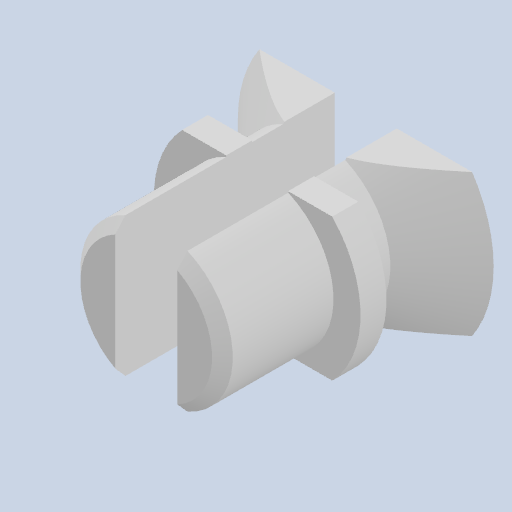
# Autodesk Inventor part: middle_gear_vtulka
Saved by Autodesk Inventor 2022 (Build 260153000, 153)
## iProperties
Created: 2024-12-03
Part Number: middle_gear_vtulka
Material: Типовые
Document SubType Name: Modeling
Designer: Andrey
Density: 1 g/cm^3
Appearance: По умолчанию
Author: Andrey
Autodesk Inventor part; units mm, degrees
ref_plane "YZ Plane" through (0, 0, 0) normal (1, 0, 0) x (0, 1, 0)
ref_plane "XZ Plane" through (0, 0, 0) normal (0, 1, 0) x (-1, 0, 0)
ref_plane "XY Plane" through (0, 0, 0) normal (0, 0, 1) x (1, 0, 0)
sketch "Эскиз1" plane through (0, 0, 0) normal (0, 1, 0) x (-1, 0, 0)
  line L0 (-19.5644, -4.2) -> (17.0679, -4.2) projected
  line L1 (-19.5644, -1.2) -> (17.0679, -1.2) projected
  line L2 (-4.6407, 3.8947) -> (-2.8372, 3.8947) projected
  line L3 (2.3395, 3.8947) -> (4.1648, 3.8947) projected
  line L4 (-7.157, -1) -> (5.9403, -1) projected
  line L5 (8.7851, 3.8947) -> (-8.7851, 3.8947)
  line L6 (4, 0) -> (-4, 0) projected
  line L7 (2.95, 0) -> (-2.95, 0)
  line L8 (2.95, -4.2) -> (2.95, 3.8947)
  line L9 (-2.95, -4.2) -> (-2.95, 3.8947)
  line L10 (2.95, -1.2) -> (4, -1.2)
  line L11 (4, 0) -> (4, -1.2)
  line L12 (-4, 0) -> (-4, -1.2)
  line L13 (-2.95, 3.8947) -> (-2.55, 4.2947)
  line L14 (-2.95, 3.8947) -> (-2.3843, 3.8947) construction
  line L15 (0, 4.2947) -> (-2.55, 4.2947)
  line L16 (0, 4.2947) -> (0, 3.8947)
  line L17 (0, 0) -> (0, 3.8947)
  line L18 (0, 4.2947) -> (-1.2, 4.2947)
  line L19 (-1.2, 4.2947) -> (-1.2, -4.2)
  line L20 (-2.95, -1.2) -> (-2.95, -4.2)
  line L21 (-2.95, -2.2) -> (-4.95, -4.2)
  line L22 (-2.95, -4.2) -> (-4.95, -4.2)
  point P0 (-4, -1)
  point P1 (-2.95, -1)
  dimension "d0" = 5.9
  dimension "d1" = 45
  dimension "d2" = 0.4
  dimension "d3" = 1.2
  dimension "d5" = 45
  dimension "d6" = 2
  constraints: 34 end point, 18 point on line, 7 perpendicular, 4 midpoint, 3 collinear, 3 horizontal, 1 equal length
  measures "d0" distance of L7.start L7.end
  measures "d1" angle of L14 L13
  measures "d2" distance of L15.start L16.end
  measures "d3" distance of L15.start L18.end
  measures "d5" angle of L20 L21
  measures "d6" distance of L9.start L21.end
revolve "Вращение1" add sketch "Эскиз1" angle 360 about axis through (0, 0, 0) along (0, 0, 1) contours L21 L9 L0 | L9 L1 L19 L0 | L9 L4 L19 L1 | L9 L6 L19 L4 | L4 L12 L6 L9 | L9 L2 L5 L19 L6 | L13 L15 L19 L5 L2
sketch "Эскиз3" plane through (0, 0, 4.2947) normal (0, 0, 1) x (1, 0, 0)
  line L0 (-1.2, 4.95) -> (1.2, 4.95)
  line L1 (1.2, 4.95) -> (1.2, -4.95)
  line L2 (1.2, -4.95) -> (-1.2, -4.95)
  line L3 (-1.2, -4.95) -> (-1.2, 4.95)
  circle A0 centre (0, 0) radius 4.95 projected
  circle A1 centre (0, 0) radius 1.2 projected
  circle A2 centre (0, 0) radius 2.75
  line L4 (-4.1158, 2.75) -> (4.1158, 2.75)
  line L5 (-4.1158, -2.75) -> (4.1158, -2.75)
  point P0 (0, 0)
  point P1 (1.2, -2.75)
  point P2 (1.2, -4.8023)
  point P3 (-1.2, -2.75)
  point P4 (-1.2, -4.8023)
  point P5 (1.2, 2.75)
  point P6 (1.2, 4.8023)
  point P7 (-1.2, 2.75)
  point P8 (-1.2, 4.8023)
  dimension "d16" = 5.5
  constraints: 12 end point, 6 tangent, 4 point on circle, 3 horizontal, 2 parallel, 1 centre point, 1 coincident, 1 perpendicular
  measures "d16" diameter of A2
extrude "Выдавливание3" cut sketch "Эскиз3" against normal blind 12 contours L0 A0 L3 | L0 L1 A0 | A0 L1 L4 L3 | L3 L4 A0 | A0 L4 L1 | L4 A2 L3 | L1 A2 L4 | A2 L1 A1 L3 | L5 L3 A0 | A1 L1 A2 L3 | A1 | A2 L5 L3 | A0 L2 L3 | L3 L5 L1 A0 | A0 L1 L5 | A2 L1 L5 | A0 L1 L2
